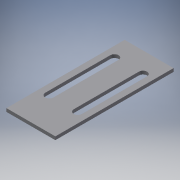
# Autodesk Inventor part: Motor holder slider
Saved by Autodesk Inventor 2018 (Build 220112000, 112)
## iProperties
Created: 2018-08-14
Part Number: Motor holder slider
Material: Generic
Document SubType Name: Modeling
Designer: ruben
Density: 1 g/cm^3
Sheet Metal Rule: Default_mm
Appearance: Default
Author: ruben
Autodesk Inventor part; units mm, degrees
ref_plane "YZ Plane" through (0, 0, 0) normal (1, 0, 0) x (0, 1, 0)
ref_plane "XZ Plane" through (0, 0, 0) normal (0, 1, 0) x (-1, 0, 0)
ref_plane "XY Plane" through (0, 0, 0) normal (0, 0, 1) x (1, 0, 0)
sketch "Sketch3" plane through (0, 0, 0) normal (0, 0, 1) x (1, 0, 0)
  line L0 (-101.5, 0) -> (101.5, 0) projected
  line L1 (0, -42) -> (0, 42) projected
  line L2 (-72.5, -30) -> (72.5, -30)
  line L3 (72.5, -30) -> (72.5, 30)
  line L4 (72.5, 30) -> (-72.5, 30)
  line L5 (-72.5, 30) -> (-72.5, -30)
  line L6 (-72.5, -30) -> (72.5, 30) construction
  line L7 (72.5, -30) -> (-72.5, 30) construction
  line L8 (-47.5, 17.5) -> (32.5, 17.5) construction
  line L9 (-47.5, 12.5) -> (32.5, 12.5)
  line L10 (32.5, 22.5) -> (-47.5, 22.5)
  arc A0 (-47.5, 22.5) -> (-47.5, 12.5) centre (-47.5, 17.5) ccw
  arc A1 (32.5, 12.5) -> (32.5, 22.5) centre (32.5, 17.5) ccw
  line L11 (-49.3038, -17.5) -> (32.5, -17.5) construction
  line L12 (-47.5, -22.5) -> (32.5, -22.5)
  line L13 (32.5, -12.5) -> (-47.5, -12.5)
  arc A2 (-47.5, -12.5) -> (-47.5, -22.5) centre (-47.5, -17.5) ccw
  arc A3 (32.5, -22.5) -> (32.5, -12.5) centre (32.5, -17.5) ccw
  point P0 (0, 0)
  dimension "d0" = 145
  dimension "d1" = 60
  dimension "d2" = 10
  dimension "d3" = 10
  dimension "d4" = 35
  dimension "d9" = 32.5
  dimension "d10" = 32.5
  dimension "d11" = 47.5
  dimension "d12" = 47.5
  constraints: 26 end point, 8 point on circle, 8 tangent, 5 parallel, 4 centre point, 2 horizontal, 2 midpoint, 2 point on line, 1 perpendicular, 1 other
  measures "d0" distance of L4.end L3.end
  measures "d1" distance of L3.end L2.end
  measures "d2" diameter of A1
  measures "d3" diameter of A3
  measures "d4" distance between parallel lines of L11 L8
  measures "d9" distance from line of L8.end L1
  measures "d10" distance from line of L11.end L1
  measures "d11" distance from line of L1 A0.centre
  measures "d12" distance from line of L1 A2.centre
extrude "Extrusion1" add sketch "Sketch3" along normal blind 4 contours L5 L4 L1 L10 A0 L9 L0 | L0 L1 L13 A2 L12 L2 L5 | L1 L9 A1 L10 L4 L3 L0 | L0 L3 L2 L1 L12 A3 L13
equation "\"d3\" = d2"
equation "\"d10\" = d9"
equation "\"d12\" = d11"
equation "\"BendRadius\" = Thickness"
equation "\"BendReliefWidth\" = Thickness"
equation "\"BendReliefDepth\" = 0.5 * Thickness"
equation "\"CornerReliefSize\" = 4 * Thickness"
equation "\"MinimumRemnant\" = 2 * Thickness"
equation "\"TransitionRadius\" = BendRadius"
equation "\"JacobiRadiusSize\" = BendRadius"
equation "\"GapSize\" = Thickness"
equation "\"Thickness\" = 0.5"
body "Solid1"
